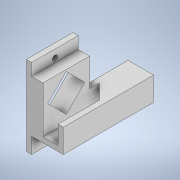
# Autodesk Inventor part: linear motion motor and gearbox holder
Saved by Autodesk Inventor 2022 (Build 260153000, 153)
## iProperties
Created: 2021-10-31
Part Number: linear motion motor and gearbox holder
Material: Generic
Document SubType Name: Modeling
Designer: alecw
Density: 1 g/cm^3
Appearance: Default
Author: alecw
Autodesk Inventor part; units mm, degrees
ref_plane "YZ Plane" through (0, 0, 0) normal (1, 0, 0) x (0, 1, 0)
ref_plane "XZ Plane" through (0, 0, 0) normal (0, 1, 0) x (-1, 0, 0)
ref_plane "XY Plane" through (0, 0, 0) normal (0, 0, 1) x (1, 0, 0)
sketch "Sketch2" plane through (0, 0, 0) normal (1, 0, 0) x (0, 1, 0)
  line L0 (0, 0) -> (14, 0)
  line L1 (14, 0) -> (16.5, 0)
  line L2 (14, 0) -> (11.5, 0)
  line L3 (14, 0) -> (28, 0)
  line L4 (14, 0) -> (-8.55, 0)
  circle A0 centre (14, 0) radius 2.75
  line L5 (-8.55, 0) -> (-8.55, 8.8)
  line L6 (-8.55, 0) -> (-8.55, -8.8)
  line L7 (0, 0) -> (0, -13.3)
  line L8 (0, -13.3) -> (6.5, -13.3)
  line L9 (0, 0) -> (0, 13.3)
  line L10 (28, 0) -> (29.5, 0)
  line L11 (29.5, 0) -> (32.5, 0)
  line L12 (-10.05, 10.3) -> (-13.05, 10.3)
  line L13 (-13.05, 10.3) -> (-13.05, 13.3)
  line L14 (-13.05, 13.3) -> (-10.05, 13.3)
  line L15 (-10.05, 13.3) -> (-10.05, 10.3)
  line L16 (-10.05, -10.3) -> (-13.05, -10.3)
  line L17 (-13.05, -10.3) -> (-13.05, -13.3)
  line L18 (-13.05, -13.3) -> (-10.05, -13.3)
  line L19 (-10.05, -13.3) -> (-10.05, -10.3)
  line L20 (-13.05, -13.3) -> (32.5, -13.3)
  line L21 (32.5, -13.3) -> (32.5, 13.3)
  line L22 (32.5, 13.3) -> (-13.05, 13.3)
  line L23 (-13.05, 13.3) -> (-13.05, -13.3)
  line L24 (9.5, 13.3) -> (-3, 13.3)
  circle A1 centre (14, 0) radius 7.5
  line L25 (28, 0) -> (25.6, 0)
  line L26 (25.6, 0) -> (25.6, -2.4)
  line L27 (25.6, 2.4) -> (25.6, -2.4)
  line L28 (25.6, 13.3) -> (25.6, -13.3)
  line L29 (32.5, 0) -> (32.5, -3)
  line L30 (28, -1.5) -> (28, -4.5)
  line L31 (28, 1.5) -> (28, 4.5)
  line L32 (32.5, 4.5) -> (25.6, 4.5)
  line L33 (25.6, 4.5) -> (25.6, -4.5)
  line L34 (25.6, -4.5) -> (32.5, -4.5)
  line L35 (32.5, -4.5) -> (32.5, 4.5)
  line L36 (0, -13.3) -> (0, -38.3)
  line L37 (0, -38.3) -> (6.5, -38.3)
  line L38 (6.5, -13.3) -> (9.5, -13.3)
  line L39 (9.5, -13.3) -> (9.5, -38.3)
  line L40 (9.5, -38.3) -> (6.5, -38.3)
  line L41 (6.5, -38.3) -> (6.5, -13.3)
  line L42 (0, -13.3) -> (-3, -13.3)
  line L43 (-3, -13.3) -> (-3, -38.3)
  line L44 (-3, -38.3) -> (0, -38.3)
  line L45 (0, -38.3) -> (0, -13.3)
  line L46 (9.5, -13.3) -> (6.5, -13.3)
  line L47 (6.5, -13.3) -> (6.5, -10.3)
  line L48 (6.5, -10.3) -> (9.5, -10.3)
  line L49 (9.5, -10.3) -> (9.5, -13.3)
  line L50 (-3, -13.3) -> (-3, 13.3)
  line L51 (-7.05, 8.8) -> (-5.05, 8.8)
  line L52 (-4.05, 13.3) -> (-4.05, -13.3)
  line L53 (9.5, -10.3) -> (9.5, 13.3)
  line L54 (6.5, -10.3) -> (6.5, 13.3)
  line L55 (25.6, -7.5) -> (0, -7.5)
  line L56 (25.6, 7.5) -> (0, 7.5)
  line L57 (14, 0) -> (19.3033, -5.3033)
  line L58 (14, 0) -> (21.5, 0) construction
  line L59 (19.3033, -5.3033) -> (14, -10.6066)
  line L60 (14, -10.6066) -> (24.6066, 0)
  line L61 (14, -10.6066) -> (3.3934, 0)
  line L62 (24.6066, 0) -> (14, 10.6066)
  line L63 (14, 10.6066) -> (3.3934, 0)
  line L64 (0, 13.3) -> (-1, 13.3)
  line L65 (-1, 13.3) -> (-1, -38.3)
  line L66 (-3, -38.3) -> (-4.05, -38.3)
  line L67 (-4.05, -38.3) -> (-4.05, -13.3)
  line L68 (25.6, 0) -> (27.6, 0)
  line L69 (25.6, 0) -> (27.6, 0)
  line L70 (27.6, 0) -> (29.1, 0)
  line L71 (29.1, 0) -> (27.1, 0)
  circle A2 centre (28, 0) radius 1.5
  circle A3 centre (-7.05, 8.8) radius 1.5
  circle A4 centre (-7.05, -8.8) radius 1.5
  point P0 (-3, -13.3)
  point P1 (6.5, 10.3)
  point P2 (6.5, -7.5)
  point P3 (6.5, 7.5)
  point P4 (6.5, -3.1066)
  point P5 (10.8934, -7.5)
  point P6 (6.5, 3.1066)
  point P7 (10.8934, 7.5)
  point P8 (17.1066, -7.5)
  point P9 (17.1066, 7.5)
  dimension "d30" = 15
  dimension "d8" = 14
  dimension "d9" = 2.5
  dimension "d10" = 2.5
  dimension "d11" = 14
  dimension "d12" = 22.55
  dimension "d14" = 5.5
  dimension "d15" = 8.8
  dimension "d19" = 13.3
  dimension "d23" = 3
  dimension "d24" = 3
  dimension "d25" = 3
  dimension "d26" = 3
  dimension "d27" = 3
  dimension "d39" = 3
  dimension "d42" = 25
  dimension "d43" = 6.5
  dimension "d44" = 3
  dimension "d45" = 3
  dimension "d46" = 3
  dimension "d47" = 2
  dimension "d55" = 45
  dimension "d58" = 15
  dimension "d64" = 1
  dimension "d65" = 2
  dimension "d66" = 1.5
  dimension "d68" = 2
  dimension "d70" = 3
  dimension "d71" = 3
  constraints: 144 end point, 27 point on line, 16 horizontal, 16 parallel, 15 perpendicular, 6 coincident, 5 vertical, 3 centre point, 3 equal length, 1 collinear, 1 vertical alignment, 6 other
  measures "d8" distance of L0.start L0.end
  measures "d9" distance of L0.end L1.end
  measures "d10" distance of L0.end L2.end
  measures "d11" distance of L0.end L3.end
  measures "d12" distance of L0.end L4.end
  measures "d14" diameter of A0
  measures "d15" distance of L4.end L5.end
  measures "d19" distance of L0.start L7.end
  measures "d23" distance of L11.start L11.end
  measures "d24" distance of L13.end L14.end
  measures "d25" distance of L12.end L13.end
  measures "d26" distance of L18.end L17.end
  measures "d27" distance of L17.end L16.end
  measures "d39" distance of L11.end L29.end
  measures "d42" distance of L7.end L36.end
  measures "d43" distance of L36.end L37.end
  measures "d44" distance of L39.end L40.end
  measures "d45" distance of L47.end L48.end
  measures "d46" distance of L46.end L47.end
  measures "d47" distance of L51.start L51.end
  measures "d55" angle of L57 L58
  measures "d58" distance of L60.end L62.end
  measures "d64" distance of L9.end L64.end
  measures "d65" distance of L25.end L68.end
  measures "d66" distance of L68.end L70.end
  measures "d68" distance of L71.start L71.end
  measures "d70" diameter of A3
  measures "d71" diameter of A4
extrude "Extrusion1" add sketch "Sketch2" along normal blind 8.6 contours L65 L20 L50 L4 | L4 L50 L22 L65 | L50 L20 L52 L4 | L4 L52 L22 L50 | L65 L44 L43 L20 | L43 L66 L67 L20 | L47 L48 L49 L20 | L20 L39 L40 L41
extrude "Extrusion2" add sketch "Sketch2" against normal blind 9.5 contours L9 L56 L54 L63 L0 | L7 L20 L65 L4 | L0 L61 L54 L55 L7 | L4 L65 L22 L9 | L65 L20 L50 L4 | L4 L50 L22 L65 | L55 L54 L47 L8 L7 | L9 L22 L54 L56 | L61 L53 L55 L54 | L54 L56 L53 L63 | L50 L20 L52 L4 | L4 L52 L22 L50 | L55 L53 L48 L54 | L54 L22 L53 L56 | L47 L48 L49 L20 | L55 L61 L59 L28 L20 L49 L53 | L53 L61 L55 | L56 L63 L53 | L53 L22 L28 L56 L62 L63 | L60 L3 L26 L28 L55 L59 | L62 L56 L28 L27 L3
extrude "Extrusion3" add sketch "Sketch2" along normal blind 3 from surface at -9.5 contours L52 L20 L19 L16 L23 L12 L15 L22 | L15 L12 L13 L14 | L18 L17 L16 L19 | L28 L34 L21 L20 | L22 L21 L32 L28 | L34 L30 A2 L11 L21 | L28 L26 L3 A2 L30 L34 | L21 L11 A2 L31 L32 | L32 L31 A2 L3 L27 L28
extrude "Extrusion4" add sketch "Sketch2" along normal blind 3 from surface at 8.6 contours L9 L56 L54 L63 L0 | L7 L20 L65 L4 | L0 L61 L54 L55 L7 | L4 L65 L22 L9 | L63 L54 L0 | L0 L54 L61 | L65 L20 L50 L4 | L4 L50 L22 L65 | L55 L54 L47 L8 L7 | L9 L22 L54 L56 | A1 L53 L0 | L54 L63 A1 | L0 L53 A1 | A1 L61 L54 | L61 L53 L55 L54 | L54 L56 L53 L63 | L50 L20 L52 L4 | L4 L52 L22 L50 | L65 L44 L43 L20 | L20 L36 L44 L65 | L8 L41 L37 L36 | L55 L53 L48 L54 | L54 L22 L53 L56 | L63 L53 A1 | A1 L53 L61 | L43 L66 L67 L20 | L47 L48 L49 L20 | L20 L39 L40 L41
sketch "Sketch3" plane through (0, 9.5, -13.3) normal (0, 1, 0) x (1, 0, 0)
  line L0 (0, -3) -> (8.6, -3) projected
  line L1 (8.6, -3) -> (0, 5.6)
  line L2 (0, 25) -> (0, 0) projected
  line L3 (8.6, -3) -> (20.7622, -3) construction
  line L4 (0, 5.6) -> (0, -3)
  line L5 (0, 0) -> (0, -26.6) projected
  line L6 (8.6, -3) -> (0, -3)
  point P0 (0, -13.3)
  point P1 (0, 0)
  dimension "d59" = 135
  constraints: 8 end point, 1 collinear, 1 equal length, 1 horizontal, 1 perpendicular, 1 point on line
  measures "d59" angle of L3 L1
extrude "Extrusion5" cut sketch "Sketch3" against normal up to next
extrude "Extrusion6" add sketch "Sketch2" against normal blind 3 contours L65 L44 L43 L20 | L20 L36 L44 L65 | L8 L41 L37 L36 | L43 L66 L67 L20 | L20 L39 L40 L41
body "Solid1"
